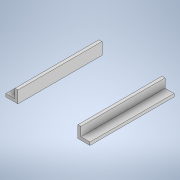
# Autodesk Inventor part: Arm holder
Saved by Autodesk Inventor 2022 (Build 260153000, 153)
## iProperties
Created: 2023-01-19
Part Number: Arm holder
Material: Generic
Document SubType Name: Modeling
Designer: s135320
Density: 1 g/cm^3
Appearance: Default
Author: s135320
Autodesk Inventor part; units mm, degrees
ref_plane "YZ Plane" through (0, 0, 0) normal (1, 0, 0) x (0, 1, 0)
ref_plane "XZ Plane" through (0, 0, 0) normal (0, 1, 0) x (-1, 0, 0)
ref_plane "XY Plane" through (0, 0, 0) normal (0, 0, 1) x (1, 0, 0)
sketch "Sketch1" plane through (0, 0, 0) normal (0, 0, 1) x (1, 0, 0)
  line L0 (0, 0) -> (-12.7, 0)
  line L1 (-12.7, 0) -> (-12.7, 12.7)
  line L2 (-12.7, 12.7) -> (0, 12.7)
  line L3 (0, 12.7) -> (0, 0)
  line L4 (-12.7, 12.7) -> (-3.175, 12.7)
  line L5 (-3.175, 12.7) -> (-3.175, 3.175)
  line L6 (-3.175, 3.175) -> (-12.7, 3.175)
  line L7 (-12.7, 3.175) -> (-12.7, 12.7)
  line L8 (63.5, 0) -> (76.2, 0)
  line L9 (76.2, 0) -> (76.2, 12.7)
  line L10 (76.2, 12.7) -> (63.5, 12.7)
  line L11 (63.5, 12.7) -> (63.5, 0)
  line L12 (76.2, 12.7) -> (66.675, 12.7)
  line L13 (66.675, 12.7) -> (66.675, 3.175)
  line L14 (66.675, 3.175) -> (76.2, 3.175)
  line L15 (76.2, 3.175) -> (76.2, 12.7)
  point P0 (-3.175, 12.7)
  dimension "d0" = 12.7
  dimension "d1" = 12.7
  dimension "d2" = 3.175
  dimension "d3" = 3.175
  dimension "d4" = 12.7
  dimension "d5" = 12.7
  dimension "d6" = 3.175
  dimension "d7" = 3.175
  dimension "d8" = 63.5
  constraints: 32 end point, 8 parallel, 4 horizontal, 4 perpendicular
  measures "d0" distance of L1.end L2.end
  measures "d1" distance of L0.end L1.end
  measures "d2" distance between parallel lines of L5 L3
  measures "d3" distance between parallel lines of L0 L6
  measures "d4" distance of L10.end L9.end
  measures "d5" distance of L9.end L8.end
  measures "d6" distance between parallel lines of L11 L13
  measures "d7" distance between parallel lines of L8 L14
  measures "d8" distance between parallel lines of L11 L3
extrude "Extrusion1" add sketch "Sketch1" along normal blind 88.9 contours L0 L1 L6 L5 L2 L3 | L11 L10 L13 L14 L9 L8
body "Solid1"
